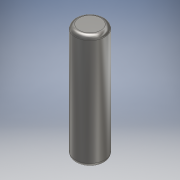
# Autodesk Inventor part: pin 1.5x5.8
Saved by Autodesk Inventor 2017 (Build 210142000, 142)
## iProperties
Created: 2018-09-03
Part Number: pin 1.5x5.8
Material: Stainless Steel
Document SubType Name: Modeling
Designer: jakub.tomczynski
Density: 8 g/cm^3
Appearance: Semi-Polished
Author: jakub.tomczynski
Autodesk Inventor part; units mm, degrees
ref_plane "YZ Plane" through (0, 0, 0) normal (1, 0, 0) x (0, 1, 0)
ref_plane "XZ Plane" through (0, 0, 0) normal (0, 1, 0) x (-1, 0, 0)
ref_plane "XY Plane" through (0, 0, 0) normal (0, 0, 1) x (1, 0, 0)
sketch "Sketch1" plane through (0, 0, 0) normal (0, 0, 1) x (1, 0, 0)
  circle A0 centre (0, 0) radius 0.75
  dimension "d0" = 1.5
  constraints: 1 centre point, 1 coincident
  measures "d0" diameter of A0
extrude "Extrusion1" add sketch "Sketch1" along normal mid plane 5.8
fillet "Fillet1" radius 0.2 2 edges at (-0.75, 0, 2.9) (-0.75, 0, -2.9)
body "Solid1"
